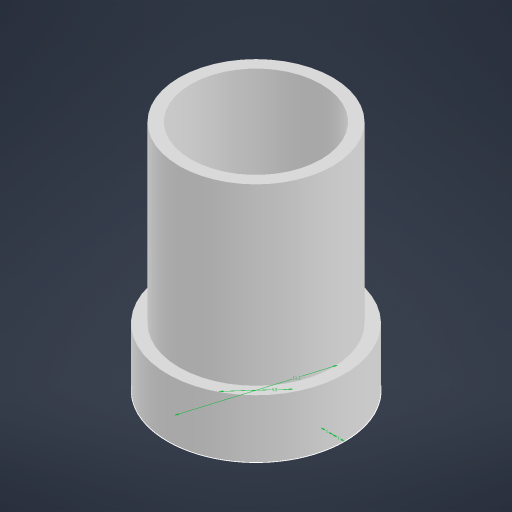
# Autodesk Inventor part: button middle part 2
Saved by Autodesk Inventor 2024.1 (Build 281209000, 209)
## iProperties
Created: 2025-01-09
Part Number: button middle part 2
Material: Generic
Document SubType Name: Modeling
Designer: Vibhu Iyer
Density: 1 g/cm^3
Appearance: Default
Author: Vibhu Iyer
Autodesk Inventor part; units mm, degrees
ref_plane "YZ Plane" through (0, 0, 0) normal (1, 0, 0) x (0, 1, 0)
ref_plane "XZ Plane" through (0, 0, 0) normal (0, 1, 0) x (-1, 0, 0)
ref_plane "XY Plane" through (0, 0, 0) normal (0, 0, 1) x (1, 0, 0)
sketch "Sketch1" plane through (0, 0, 0) normal (0, 1, 0) x (-1, 0, 0)
  circle A0 centre (0, 0) radius 5.6
  circle A1 centre (0, 0) radius 2.25
  circle A2 centre (0, 0) radius 6.6
  circle A3 centre (0, 0) radius 7.6
  dimension "d0" = 11.2
  dimension "d1" = 4.5
  dimension "d6" = 1
  dimension "d7" = 1
  constraints: 4 centre point, 2 coincident
  measures "d0" diameter of A0
  measures "d1" diameter of A1
  measures "d6" radial gap between concentric circles of A0 A2
  measures "d7" radial gap between concentric circles of A2 A3
extrude "Extrusion1" add sketch "Sketch1" along normal blind 5 contours A0 | A2 | A3
extrude "Extrusion3" add sketch "Sketch1" along normal blind 15 from surface at 5 contours A2
sketch "Sketch4" plane through (0, 5, 0) normal (0, 1, 0) x (1, 0, 0)
  circle A0 centre (0, 3.925) radius 1.25
  circle A1 centre (0, 0) radius 2.25 projected
  line L0 (0, 2.25) -> (0, 5.6) construction
  circle A2 centre (0, 0) radius 5.6 projected
  dimension "d19" = 2.5
  constraints: 3 vertical alignment, 2 end point, 1 centre point, 1 coincident, 1 midpoint, 1 vertical, 2 other
  measures "d19" diameter of A0
extrude "Extrusion5" cut sketch "Sketch4" against normal up to surface (5 mm away) contours A0
body "Solid1"
